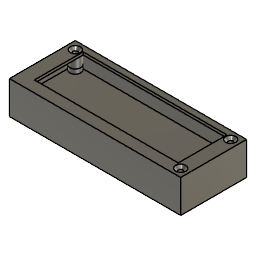
RC1602E_display_case (Autodesk Fusion 360 design; units mm, degrees)
Autodesk Fusion 360 part; units mm, degrees
sketch "Sketch1" plane through (0, 0, 0) normal (0, 0, 1) x (1, 0, 0)
  line L0 (0, 0) -> (80, 0)
  line L1 (80, 0) -> (80, 36)
  line L2 (80, 36) -> (0, 36)
  line L3 (0, 36) -> (0, 0)
  line L4 (0, 0) -> (122, 0)
  line L5 (122, 0) -> (122, 44)
  line L6 (122, 44) -> (0, 44)
  line L7 (0, 44) -> (0, 0)
  line L8 (-0.4, -0.4) -> (122.4, -0.4)
  line L9 (122.4, -0.4) -> (122.4, 44.4)
  line L10 (122.4, 44.4) -> (-0.4, 44.4)
  line L11 (-0.4, 44.4) -> (-0.4, -0.4)
  line L12 (-2.4, -2.4) -> (124.4, -2.4)
  line L13 (124.4, -2.4) -> (124.4, 46.4)
  line L14 (124.4, 46.4) -> (-2.4, 46.4)
  line L15 (-2.4, 46.4) -> (-2.4, -2.4)
  circle A0 centre (118.5, 40.5) radius 1.75
  circle A1 centre (118.5, 3.5) radius 1.75
  circle A2 centre (3.5, 40.5) radius 1.75
  circle A3 centre (3.5, 40.5) radius 4
  circle A4 centre (118.5, 40.5) radius 4
  circle A5 centre (118.5, 3.5) radius 4
  line L16 (7.8, 42) -> (114.2, 42)
  line L17 (114.2, 42) -> (114.2, 6)
  line L18 (114.2, 6) -> (7.8, 6)
  line L19 (7.8, 6) -> (7.8, 42)
  point P0 (10.98, 2.5)
  dimension "d1" = 36
  dimension "d2" = 80
  dimension "d5" = 2.5
  dimension "d6" = 10.98
  dimension "d7" = 122
  dimension "d8" = 44
  dimension "d9" = 0.4
  dimension "d10" = 2
  dimension "d11" = 3.5
  dimension "d12" = 3.5
  dimension "d14" = 3.5
  dimension "d15" = 3.5
  dimension "d16" = 3.5
  dimension "d17" = 3.5
  dimension "d18" = 3.5
  dimension "d19" = 3.5
  dimension "d20" = 3.5
  dimension "d23" = 8
  dimension "d24" = 8
  dimension "d25" = 8
  dimension "d27" = 2
  dimension "d28" = 36
  dimension "d29" = 7.8
  dimension "d30" = 106.4
  constraint horizontal L0
  constraint vertical L1
  constraint horizontal L2
  constraint vertical L3
  constraint coincident L0.start L3.end
  constraint horizontal L4
  constraint vertical L5
  constraint horizontal L6
  constraint vertical L7
  constraint concentric A2 A3
  constraint concentric A0 A4
  constraint concentric A1 A5
  constraint horizontal L16
  constraint vertical L17
  constraint horizontal L18
  constraint vertical L19
  measures "d1" distance of L0 L2
  measures "d2" distance of L1 L3
  measures "d5" distance of L0 P0
  measures "d6" distance of L3 P0
  measures "d7" distance of L5 L7
  measures "d8" distance of L4 L6
  measures "d11" diameter of A0
  measures "d12" diameter of A1
  measures "d14" diameter of A2
  measures "d15" distance of L3 A2.centre
  measures "d16" distance of L6 A2.centre
  measures "d17" distance of L6 A0.centre
  measures "d18" distance of L5 A0.centre
  measures "d19" distance of L5 A1.centre
  measures "d20" distance of L4 A1.centre
  measures "d23" diameter of A3
  measures "d24" diameter of A4
  measures "d25" diameter of A5
  measures "d27" distance of L6 L16
  measures "d28" distance of L16 L18
  measures "d29" distance of L7 L19
  measures "d30" distance of L17 L19
extrude "Extrude4" add sketch "Sketch1" along normal blind 9.6 contours L0 L1 L2 L3 L4 L7 L18 L19 | L0 L3 L4 L7 L8 L11 A3 A5 | L1 L2 L4 L5 L6 L7 A3 A4 A5 L16 L17 L18 L19 | L1 L2 L18 L19 | L1 L2 L16 L17 L18 L19 | L4 L5 A5 | L4 L8 A5 | L7 L11 A3 | L6 L7 A3 | L4 L5 A5 | L4 L5 L8 L9 A5 | L5 L9 A5 | L5 L9 A4 A5 | L8 A5 | L6 L7 L10 L11 A3 | L6 L7 A3 | L11 A3 | L5 L6 A4 | L5 L9 A4 | L9 A5 | L6 L10 A3 | L6 L10 A3 A4 | L5 L6 A4 | L5 L6 L9 L10 A4 | L6 L10 A4 | L9 A4 | L10 A3 | L10 A4 | L12 L13 L14 L15 makes body 1
extrude "Extrude5" cut sketch "Sketch1" along normal blind 9.6 contours L1 L2 L18 L19 | L1 L2 L16 L17 L18 L19 bodies 1
extrude "Extrude6" cut sketch "Sketch1" along normal blind 7.6 contours L0 L1 L2 L3 L4 L7 L18 L19 | L0 L3 L4 L7 L8 L11 A3 A5 | L1 L2 L4 L5 L6 L7 A3 A4 A5 L16 L17 L18 L19 | L4 L5 A5 | L4 L5 L8 L9 A5 | L5 L9 A4 A5 | L6 L7 L10 L11 A3 | L6 L7 A3 | L6 L10 A3 A4 | L5 L6 A4 | L5 L6 L9 L10 A4 picked at (121.4115, 0.3254) picked at (0.3254, 43.4115) picked at (121.4115, 43.6746) bodies 1
extrude "Extrude7" add sketch "Sketch1" against normal blind 14.8 contours L8 A5 | L11 A3 | L9 A5 | L9 A4 | L10 A3 | L10 A4 | L12 L13 L14 L15 bodies 1
extrude "Extrude8" add sketch "Sketch1" against normal blind 5.3 separate body contours L0 L1 L2 L3 L4 L7 L18 L19 | L1 L2 L4 L5 L6 L7 A3 A4 A5 L16 L17 L18 L19 | L1 L2 L18 L19 | L1 L2 L16 L17 L18 L19 | L4 L5 A5 | L6 L7 A3 | L4 L5 A5 | L6 L7 A3 | L5 L6 A4 | L5 L6 A4 makes body 2
extrude "Extrude9" cut sketch "Sketch1" against normal blind 3.3 contours L0 L1 L2 L3 L4 L7 L18 L19 | L1 L2 L4 L5 L6 L7 A3 A4 A5 L16 L17 L18 L19 | L1 L2 L18 L19 | L1 L2 L16 L17 L18 L19 | L4 L5 A5 | L6 L7 A3 | L5 L6 A4 picked at (121.4115, 0.3254) picked at (0.3254, 43.4115) picked at (121.4115, 43.6746) bodies 2
sketch "Sketch2" plane through (-2.4, 0, 0) normal (-1, 0, 0) x (0, -1, 0)
  line L0 (2.4, -14.8) -> (2.4, 9.6)
  line L1 (2.4, 9.6) -> (-46.4, 9.6)
  line L2 (-46.4, 9.6) -> (-46.4, -14.8)
  line L3 (-46.4, -14.8) -> (2.4, -14.8)
  line L4 (-24.1, -5) -> (-11.1, -5)
  line L5 (-11.1, -5) -> (-11.1, -13)
  line L6 (-11.1, -13) -> (-24.1, -13)
  line L7 (-24.1, -13) -> (-24.1, -5)
  line L8 (-7.5, 0) -> (0.4, 0)
  dimension "d49" = 8
  dimension "d50" = 13
  dimension "d52" = 5
  dimension "d57" = 13.5
  constraint horizontal L4
  constraint vertical L5
  constraint horizontal L6
  constraint vertical L7
  measures "d49" distance of L4 L6
  measures "d50" distance of L5 L7
  measures "d52" distance of L4 L8
  measures "d57" distance of L0 L5
extrude "Extrude10" cut sketch "Sketch2" against normal blind 2 contours L4 L5 L6 L7 bodies 1
chamfer "Chamfer1" distance 2 angle 45 3 edges at (116.8684, 41.1328, 9.6) (116.8684, 4.1328, 9.6) (1.8684, 41.1328, 9.6) tangent chain off on bodies 1
chamfer "Chamfer2" distance 1.8 angle 45 3 edges at (116.8684, 2.8672, -5.3) (116.8684, 39.8672, -5.3) (1.8684, 39.8672, -5.3) tangent chain off on bodies 2
